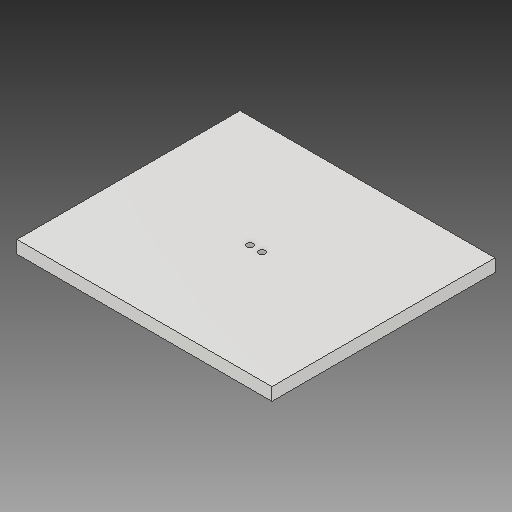
# Autodesk Inventor part: platform_top
Saved by Autodesk Inventor 2018.1 (Build 221171000, 171)
## iProperties
Created: 2017-07-26
Part Number: platform_top
Material: PVC-Piping
Document SubType Name: Modeling
Designer: Tom
Density: 1.4 g/cm^3
Appearance: Smooth - White
Mass: 3917.57 g
Surface Area: 3107.92 cm^2
Volume: 2798.27 cm^3
Author: Tom
Autodesk Inventor part; units mm, degrees
ref_plane "YZ Plane" through (0, 0, 0) normal (1, 0, 0) x (0, 1, 0)
ref_plane "XZ Plane" through (0, 0, 0) normal (0, 1, 0) x (-1, 0, 0)
ref_plane "XY Plane" through (0, 0, 0) normal (0, 0, 1) x (1, 0, 0)
sketch "Sketch1" plane through (0, 0, 0) normal (0, 0, 1) x (1, 0, 0)
  line L0 (0, 0) -> (400, 0)
  line L1 (400, 0) -> (400, 350)
  line L2 (400, 350) -> (0, 350)
  line L3 (0, 350) -> (0, 0)
  dimension "d0" = 400
  dimension "d1" = 350
  constraints: 8 end point, 2 parallel, 1 horizontal, 1 perpendicular
  measures "d0" distance of L2.end L1.end
  measures "d1" distance of L1.end L0.end
extrude "Extrusion1" add sketch "Sketch1" along normal blind 20
sketch "Sketch2" plane through (0, 0, 0) normal (0, 0, -1) x (-1, 0, 0)
  circle A0 centre (-190.475, 175) radius 3 projected
  circle A1 centre (-209.525, 175) radius 3 projected
  point P0 (0, 0)
extrude "Extrusion2" cut sketch "Sketch2" against normal blind 20
sketch "Sketch4" plane through (0, 0, 0) normal (0, 0, -1) x (-1, 0, 0)
  circle A0 centre (-190.475, 175) radius 3 construction
  circle A1 centre (-209.525, 175) radius 3 construction
  circle A2 centre (-190.475, 175) radius 5
  circle A3 centre (-209.525, 175) radius 5
  point P0 (0, 0)
  dimension "d10" = 10
  dimension "d11" = 10
  constraints: 2 centre point, 2 coincident
  measures "d10" diameter of A2
  measures "d11" diameter of A3
extrude "Extrusion4" cut sketch "Sketch4" against normal blind 6
equation "\"d0\" = maxl"
equation "\"d1\" = maxw"
equation "\"d2\" = platft"
equation "\"d4\" = platft"
equation "\"d10\" = bhd"
equation "\"d11\" = bhd"
equation "\"d12\" = bhh"
equation "\"dias\" = 8.8"
equation "\"stra1\" = 9.5"
equation "\"diab2\" = 6"
equation "\"stra\" = 25"
equation "\"db1\" = 6"
equation "\"ds1\" = 5.8"
equation "\"ds2\" = 1.6"
equation "\"ang\" = 120deg"
equation "\"db2\" = 3"
equation "\"diab3\" = 7"
equation "\"diab4\" = 3"
equation "\"dias1\" = 13.4375"
equation "\"dias3\" = 2"
equation "\"dias4\" = 4"
equation "\"t1\" = 3"
equation "\"t2\" = 3"
equation "\"t3\" = 6"
equation "\"t4\" = 6"
equation "\"t5\" = 3"
equation "\"diab1\" = 19"
equation "\"afw\" = 0.2"
equation "\"maxw\" = 350"
equation "\"lcsd\" = 19.05"
equation "\"lcwd1\" = 25"
equation "\"lch1\" = 39"
equation "\"lcwd2\" = 34"
equation "\"lcwd3\" = 43"
equation "\"dia1\" = 6"
equation "\"td\" = 18"
equation "\"bhh\" = 6"
equation "\"bhd\" = 10"
equation "\"spacert\" = 2"
equation "\"sh\" = 31"
equation "\"sw\" = 25"
equation "\"platft\" = 20"
equation "\"pvct\" = 5"
equation "\"dia3\" = 8"
equation "\"dia4\" = 11"
equation "\"tankl\" = 379"
equation "\"play\" = 9"
equation "\"holeh\" = 26"
equation "\"slack\" = 0.5"
equation "\"surroundt\" = 5"
equation "\"play2\" = 3"
equation "\"maxl\" = 400"
equation "\"diaoverflow\" = 25"
equation "\"diawater\" = 25"
equation "\"diacucl\" = 32"
equation "\"diaair\" = 32"
equation "\"diaph\" = 32"
equation "\"diasurroundhole\" = 42"
equation "\"diagrate\" = 12"
equation "\"gratespacing\" = 12.02082"
equation "\"sidedist\" = 13.9375"
equation "\"bottomdist\" = 9.6355"
equation "\"diahcl\" = 32"
equation "\"bracketwtop\" = 6"
equation "\"bracketwbottom\" = 6"
equation "\"nett\" = 1"
equation "\"nethole\" = 16"
equation "\"nettop\" = 7"
equation "\"netside\" = 3.5"
equation "\"netholespacing\" = 2"
equation "\"diaetape\" = 32"
body "Solid1"
